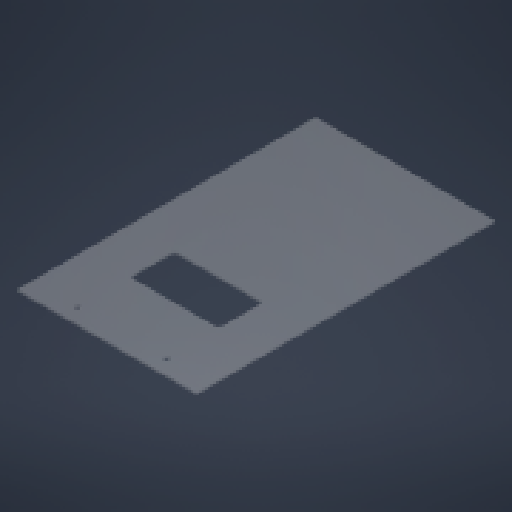
# Autodesk Inventor part: 2polycarb10x6
Saved by Autodesk Inventor 2023 (Build 270158000, 158)
## iProperties
Created: 2023-01-26
Part Number: 2polycarb10x6
Material: Polycarbonate, Clear
Document SubType Name: Modeling
Designer: Windows Macbook
Density: 1.2 g/cm^3
Appearance: Polycarbonate - Clear
Author: Windows Macbook
Autodesk Inventor part; units mm, degrees
ref_plane "YZ Plane" through (0, 0, 0) normal (1, 0, 0) x (0, 1, 0)
ref_plane "XZ Plane" through (0, 0, 0) normal (0, 1, 0) x (-1, 0, 0)
ref_plane "XY Plane" through (0, 0, 0) normal (0, 0, 1) x (1, 0, 0)
sketch "Sketch1" plane through (0, 0, 0) normal (0, 1, 0) x (-1, 0, 0)
  line L0 (-101.6, -127) -> (50.8, -127)
  line L1 (50.8, -127) -> (50.8, 127)
  line L2 (50.8, 127) -> (-101.6, 127)
  line L3 (-101.6, 127) -> (-101.6, -127)
  point P0 (0, 0)
  dimension "d0" = 152.4
  dimension "d1" = 254
  constraints: 8 end point, 2 parallel, 1 horizontal, 1 perpendicular
  measures "d0" distance of L2.end L1.end
  measures "d1" distance of L1.end L0.end
extrude "Extrusion2" add sketch "Sketch1" along normal blind 1.5875
sketch "Sketch3" plane through (0, 1.5875, 0) normal (0, 1, 0) x (1, 0, 0)
  circle A0 centre (63.5, -114.3) radius 2.1844
  circle A1 centre (-12.7, -114.3) radius 2.1844
  point P0 (0, 0)
  dimension "d13" = 4.3688
  dimension "d14" = 4.3688
  constraints: 2 centre point
  measures "d13" diameter of A0
  measures "d14" diameter of A1
hole "Hole1" at (63.5, 1.5875, 114.3) at (-12.7, 1.5875, 114.3) direction (0, -1, 0) diameter 4.3688 end through all
sketch "Sketch4" plane through (0, 0, 0) normal (0, -1, 0) x (1, 0, 0)
  line L0 (101.6, 127) -> (101.6, -127) projected
  line L1 (-50.8, -127) -> (-50.8, 127) projected
  line L2 (101.6, 50.8) -> (254, 50.8) construction
  line L3 (-12.7, 34.925) -> (-12.7, 66.675)
  line L4 (63.5, 66.675) -> (63.5, 34.925)
  line L5 (-12.7, 66.675) -> (-12.7, 69.85)
  line L6 (63.5, 73.025) -> (-12.7, 73.025)
  line L7 (-12.7, 73.025) -> (-12.7, 28.575)
  line L8 (-12.7, 28.575) -> (63.5, 28.575)
  line L9 (63.5, 28.575) -> (63.5, 73.025)
  point P0 (0, 0)
  point P1 (-12.7, 31.75)
  point P2 (63.5, 69.85)
  dimension "d24" = 76.2
  dimension "d25" = 38.1
  constraints: 16 end point, 4 point on line, 3 parallel, 2 coincident, 2 horizontal, 1 perpendicular, 1 vertical
  measures "d24" distance of L5.end point (63.5, 69.85)
  measures "d25" distance of point (-12.7, 31.75) L5.end
extrude "Extrusion5" cut sketch "Sketch4" against normal up to next
body "Solid2"
